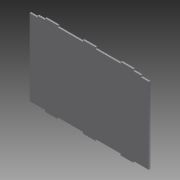
# Autodesk Inventor part: it shelf
Saved by Autodesk Inventor 2011 (Build 150239000, 239)
## iProperties
Created: 2011-09-10
Part Number: it shelf
Document SubType Name: Modeling
Designer: Matthew
Density: 1 g/cm^3
Author: Matthew
Autodesk Inventor part; units mm, degrees
ref_plane "YZ Plane" through (0, 0, 0) normal (1, 0, 0) x (0, 1, 0)
ref_plane "XZ Plane" through (0, 0, 0) normal (0, 1, 0) x (-1, 0, 0)
ref_plane "XY Plane" through (0, 0, 0) normal (0, 0, 1) x (1, 0, 0)
sketch "Sketch1" plane through (0, 0, 0) normal (0, 0, 1) x (1, 0, 0)
  line L0 (-38.1107, 23.9821) -> (441.9493, 23.9821)
  line L1 (441.9493, 23.9821) -> (441.9493, -289.7079)
  line L2 (441.9493, -289.7079) -> (-38.1107, -289.7079)
  line L3 (-38.1107, -289.7079) -> (-38.1107, 23.9821)
  line L4 (-38.1107, -289.7079) -> (227.3193, -289.7079)
  line L5 (227.3193, -289.7079) -> (176.5193, -289.7079)
  line L6 (176.5193, -289.7079) -> (176.5193, -296.0579)
  line L7 (176.5193, -296.0579) -> (227.3193, -296.0579)
  line L8 (227.3193, -296.0579) -> (227.3193, -289.7079)
  line L9 (227.3193, -289.7079) -> (328.9193, -289.7079)
  line L10 (328.9193, -289.7079) -> (74.9193, -289.7079)
  line L11 (74.9193, -289.7079) -> (24.1193, -289.7079)
  line L12 (24.1193, -289.7079) -> (24.1193, -296.0579)
  line L13 (24.1193, -296.0579) -> (74.9193, -296.0579)
  line L14 (74.9193, -296.0579) -> (74.9193, -289.7079)
  line L15 (328.9193, -289.7079) -> (379.7193, -289.7079)
  line L16 (379.7193, -289.7079) -> (379.7193, -296.0579)
  line L17 (379.7193, -296.0579) -> (328.9193, -296.0579)
  line L18 (328.9193, -296.0579) -> (328.9193, -289.7079)
  line L19 (24.1193, 23.9821) -> (74.9193, 23.9821)
  line L20 (74.9193, 23.9821) -> (74.9193, 30.3321)
  line L21 (74.9193, 30.3321) -> (24.1193, 30.3321)
  line L22 (24.1193, 30.3321) -> (24.1193, 23.9821)
  line L23 (176.5193, 23.9821) -> (227.3193, 23.9821)
  line L24 (227.3193, 23.9821) -> (227.3193, 30.3321)
  line L25 (227.3193, 30.3321) -> (176.5193, 30.3321)
  line L26 (176.5193, 30.3321) -> (176.5193, 23.9821)
  line L27 (328.9193, 23.9821) -> (379.7193, 23.9821)
  line L28 (379.7193, 23.9821) -> (379.7193, 30.3321)
  line L29 (379.7193, 30.3321) -> (328.9193, 30.3321)
  line L30 (328.9193, 30.3321) -> (328.9193, 23.9821)
  line L31 (-38.1107, 23.9821) -> (-6.1067, 23.9821)
  line L32 (-6.1067, 23.9821) -> (-6.1067, 17.3781)
  line L33 (-6.1067, 17.3781) -> (-38.1107, 17.3781)
  line L34 (-38.1107, 17.3781) -> (-38.1107, 23.9821)
  line L35 (441.9493, 23.9821) -> (409.9453, 23.9821)
  line L36 (409.9453, 23.9821) -> (409.9453, 17.3781)
  line L37 (409.9453, 17.3781) -> (441.9493, 17.3781)
  line L38 (441.9493, 17.3781) -> (441.9493, 23.9821)
  point P0 (0, 0)
  dimension "d0" = 480.06
  dimension "d1" = 313.69
  dimension "d2" = 265.43
  dimension "d3" = 50.8
  dimension "d4" = 6.35
  dimension "d5" = 101.6
  dimension "d6" = 254
  dimension "d7" = 50.8
  dimension "d8" = 50.8
  dimension "d9" = 6.35
  dimension "d10" = 32.004
  dimension "d11" = 6.604
  dimension "d12" = 32.004
  constraints: 78 end point, 18 parallel, 9 horizontal, 9 perpendicular, 6 point on line
  measures "d0" distance of L1.end L2.end
  measures "d1" distance of L0.end L1.end
  measures "d2" distance of L2.end L4.end
  measures "d3" distance of L7.end L6.end
  measures "d4" distance of L6.end L5.end
  measures "d5" distance of L4.end L9.end
  measures "d6" distance of L9.end L10.end
  measures "d7" distance of L13.end L12.end
  measures "d8" distance of L16.end L17.end
  measures "d9" distance of L20.end L19.end
  measures "d10" distance of L32.end L33.end
  measures "d11" distance of L31.end L32.end
  measures "d12" distance of L37.end L36.end
extrude "Extrusion1" add sketch "Sketch1" along normal blind 6.35 contours L0 L36 L37 L1 L2 L3 L33 L32 | L22 L21 L20 L0 | L2 L14 L13 L12 | L26 L25 L24 L0 | L2 L8 L7 L6 | L30 L29 L28 L0 | L2 L16 L17 L18
body "Solid1"
